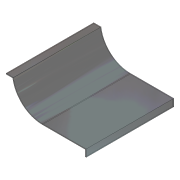
# Autodesk Inventor part: Panel_FrontVerticalConveyorShroud_Upper
Saved by Autodesk Inventor 2012 (Build 160160000, 160)
## iProperties
Created: 2012-01-26
Part Number: Panel_FrontVerticalConveyorShroud_Upper
Material: Polycarbonate, Smoke
Document SubType Name: Modeling
Designer: JesseK
Mass: 402.26 g
Surface Area: 2152.98 cm^2
Volume: 335.216 cm^3
Density: 1.2 g/cm^3
Author: JesseK
Autodesk Inventor part; units mm, degrees
ref_plane "YZ Plane" through (0, 0, 0) normal (1, 0, 0) x (0, 1, 0)
ref_plane "XZ Plane" through (0, 0, 0) normal (0, 1, 0) x (-1, 0, 0)
ref_plane "XY Plane" through (0, 0, 0) normal (0, 0, 1) x (1, 0, 0)
sketch "Sketch1" plane through (0, 0, 0) normal (0, 0, 1) x (1, 0, 0)
  arc A0 (-100.8031, -12.7) -> (0, -101.6) centre (0, 0) ccw
  line L0 (0, -101.6) -> (152.4, -101.6)
  line L1 (152.4, -101.6) -> (152.4, -127)
  line L2 (149.225, -104.775) -> (0, -104.775)
  arc A1 (-103.5654, -15.875) -> (0, -104.775) centre (0, 0) ccw
  line L3 (-100.8031, -12.7) -> (-126.2031, -12.7)
  line L4 (-126.2031, -12.7) -> (-126.2031, -15.875)
  line L5 (-126.2031, -15.875) -> (-103.5654, -15.875)
  line L6 (-126.2031, -12.7) -> (-100.8031, -12.7)
  line L7 (-100.8031, -12.7) -> (-100.8031, 0)
  line L8 (-100.8031, 0) -> (-126.2031, 0)
  line L9 (-126.2031, 0) -> (-126.2031, -12.7)
  line L10 (-100.8031, 0) -> (0, 0) construction
  line L11 (149.225, -104.775) -> (149.225, -127)
  line L12 (149.225, -127) -> (152.4, -127)
  dimension "d0" = 25.4
  dimension "d2" = 3.175
  dimension "d3" = 3.175
  dimension "d4" = 12.7
  dimension "d5" = 101.6
  dimension "d6" = 152.4
  dimension "d7" = 3.175
  dimension "d8" = 25.4
  constraints: 26 end point, 4 parallel, 4 point on circle, 3 horizontal, 2 centre point, 2 coincident, 2 collinear, 2 perpendicular, 2 tangent, 2 vertical
  measures "d0" distance of L7.end L8.end
  measures "d2" radial gap between concentric circles of A1 A0
  measures "d3" distance between parallel lines of L3 L5
  measures "d4" distance of L8.end L3.end
  measures "d5" radius of A0
  measures "d6" distance of L0.start L0.end
  measures "d7" distance of L11.end L1.end
  measures "d8" distance of L0.end L1.end
extrude "Extrusion1" add sketch "Sketch1" along normal blind 304.8 contours A0 L0 L1 L12 L11 L2 A1 L5 L4 L3
body "Solid1"
